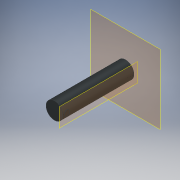
# Autodesk Inventor part: Tige d'entraintenement
Saved by Autodesk Inventor 2018 (Build 220112000, 112)
## iProperties
Created: 2017-10-08
Part Number: Tige d'entraintenement
Material: Iron, Cast
Document SubType Name: Modeling
Designer: liamg
Density: 7.15 g/cm^3
Appearance: Iron Gray
Author: liamg
Autodesk Inventor part; units mm, degrees
ref_plane "XZ Plane" through (0, 0, 0) normal (0, 1, 0) x (-1, 0, 0)
ref_plane "XY Plane" through (0, 0, 0) normal (0, 0, 1) x (1, 0, 0)
ref_plane "Work Plane1" through (46.1125, -75.7898, -8.2516) normal (0, 0, 1) x (1, 0, 0)
sketch "Sketch1" plane through (46.1125, -75.7898, -8.2516) normal (0, 0, 1) x (1, 0, 0)
  circle A0 centre (0, 0) radius 1.6 projected
  point P0 (-46.1125, 75.7898)
extrude "Extrusion1" add sketch "Sketch1" along normal blind 13.5
ref_plane "Work Plane2" through (47.7125, -75.7898, -8.2516) normal (1, 0, 0) x (0, 1, 0)
sketch "Sketch2" plane through (47.7125, -75.7898, -8.2516) normal (1, 0, 0) x (0, 1, 0)
  circle A0 centre (0.0121, 12.6933) radius 0.4995
  point P0 (75.7898, 8.2516)
  constraints: 1 centre point
extrude "Extrusion2" add sketch "Sketch2" against normal up to next
body "Solid1"
